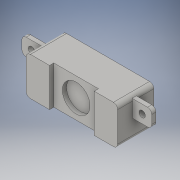
# Autodesk Inventor part: Speaker
Saved by Autodesk Inventor 2016 (Build 200138000, 138)
## iProperties
Created: 2015-10-01
Part Number: Speaker
Material: Generic
Document SubType Name: Modeling
Designer: fei
Density: 1 g/cm^3
Appearance: Default
Author: fei
Autodesk Inventor part; units mm, degrees
ref_plane "YZ Plane" through (0, 0, 0) normal (1, 0, 0) x (0, 1, 0)
ref_plane "XZ Plane" through (0, 0, 0) normal (0, 1, 0) x (-1, 0, 0)
ref_plane "XY Plane" through (0, 0, 0) normal (0, 0, 1) x (1, 0, 0)
sketch "Sketch1" plane through (0, 0, 0) normal (1, 0, 0) x (0, 1, 0)
  line L0 (228.6, 215.9) -> (-228.6, 215.9)
  line L1 (-228.6, 215.9) -> (-228.6, -215.9)
  line L2 (-228.6, -215.9) -> (228.6, -215.9)
  line L3 (228.6, -215.9) -> (228.6, 215.9)
  point P0 (0, 0)
  dimension "d0" = 431.8
  dimension "d1" = 457.2
  dimension "d2" = 215.9
  dimension "d3" = 228.6
  constraints: 8 end point, 2 parallel, 1 horizontal, 1 perpendicular
  measures "d0" distance of L2.end L0.start
  measures "d1" distance of L1.end L2.end
  measures "d2" distance from line of L2 point (0, 0)
  measures "d3" distance from line of point (0, 0) L3
extrude "Extrusion1" add sketch "Sketch1" along normal mid plane 1092.2
sketch "Sketch2" plane through (546.1, 0, 0) normal (1, 0, 0) x (0, 0, -1)
  line L0 (-38.1, 203.2) -> (12.7, 203.2)
  line L1 (12.7, 203.2) -> (12.7, 0)
  line L2 (12.7, 0) -> (-38.1, 0)
  line L3 (-38.1, 0) -> (-38.1, 203.2)
  line L4 (-215.9, 228.6) -> (-215.9, -228.6) projected
  line L5 (-215.9, 228.6) -> (215.9, 228.6) projected
  point P0 (0, 0)
  dimension "d6" = 50.8
  dimension "d7" = 203.2
  dimension "d8" = 228.6
  dimension "d9" = 25.4
  constraints: 8 end point, 2 parallel, 1 horizontal, 1 perpendicular
  measures "d6" distance of L0.start L0.end
  measures "d7" distance of L0.end L1.end
  measures "d8" distance between parallel lines of L4 L1
  measures "d9" distance between parallel lines of L5 L0
extrude "Extrusion2" add sketch "Sketch2" along normal blind 228.6
mirror "Mirror1" about plane through (0, 0, 0) normal (1, 0, 0) of "Extrusion2"
sketch "Sketch3" plane through (546.1, 0, 38.1) normal (0, 0, 1) x (1, 0, 0)
  circle A0 centre (114.3, 101.6) radius 38.1
  line L0 (0, 228.6) -> (0, -228.6) projected
  line L1 (0, 203.2) -> (228.6, 203.2) projected
  point P0 (-546.1, 0)
  dimension "d12" = 76.2
  dimension "d13" = 114.3
  dimension "d14" = 101.6
  constraints: 1 centre point
  measures "d12" diameter of A0
  measures "d13" distance from line of L0 A0.centre
  measures "d14" distance from line of A0.centre L1
extrude "Extrusion3" cut sketch "Sketch3" against normal through all
mirror "Mirror2" about plane through (0, 0, 0) normal (1, 0, 0) of "Extrusion3"
fillet "Fillet1" radius 50.8 8 edges at (774.7, 203.2, 12.7) (774.7, 0, 12.7) (546.1, 228.6, 0) (546.1, -228.6, 0) (-546.1, 228.6, 0) (-546.1, -228.6, 0) (-774.7, 203.2, 12.7) (-774.7, 0, 12.7)
sketch "Sketch4" plane through (-495.3, -228.6, 215.9) normal (0, 0, 1) x (1, 0, 0)
  circle A0 centre (495.3, 228.6) radius 165.1
  dimension "d18" = 330.2
  constraints: 1 centre point, 1 coincident
  measures "d18" diameter of A0
extrude "Extrusion4" cut sketch "Sketch4" against normal blind 101.6
sketch "Sketch5" plane through (-495.3, -228.6, 215.9) normal (0, 0, 1) x (1, 0, 0)
  line L0 (990.6, 457.2) -> (0, 457.2) projected
  line L1 (0, 0) -> (990.6, 0) projected
  line L2 (228.6, 457.2) -> (762, 457.2)
  line L3 (762, 457.2) -> (762, 0)
  line L4 (762, 0) -> (228.6, 0)
  line L5 (228.6, 0) -> (228.6, 457.2)
  line L6 (1041.4, 406.4) -> (1041.4, 50.8) projected
  line L7 (-50.8, 50.8) -> (-50.8, 406.4) projected
  point P0 (495.3, 228.6)
  dimension "d21" = 279.4
  dimension "d22" = 279.4
  constraints: 8 end point, 2 parallel, 2 point on line, 1 horizontal, 1 perpendicular
  measures "d21" distance between parallel lines of L6 L3
  measures "d22" distance between parallel lines of L7 L5
extrude "Extrusion5" cut sketch "Sketch5" against normal blind 50.8
body "Solid1"
